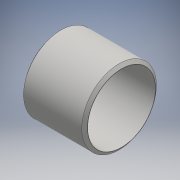
# Autodesk Inventor part: Rear Head Pipe
Saved by Autodesk Inventor 2016 (Build 200138000, 138)
## iProperties
Created: 2018-11-05
Part Number: Rear Head Pipe
Material: Steel ASTM A53 Gr.B
Document SubType Name: Modeling
Designer: asus
Density: 7.58 g/cm^3
Appearance: Plate(1)
Mass: 38975.2 g
Surface Area: 6569.07 cm^2
Volume: 5141.85 cm^3
Author: asus
Autodesk Inventor part; units mm, degrees
ref_plane "YZ Plane" through (0, 0, 0) normal (1, 0, 0) x (0, 1, 0)
ref_plane "XZ Plane" through (0, 0, 0) normal (0, 1, 0) x (-1, 0, 0)
ref_plane "XY Plane" through (0, 0, 0) normal (0, 0, 1) x (1, 0, 0)
sketch "Sketch1" plane through (0, 0, 0) normal (0, 0, 1) x (1, 0, 0)
  line L0 (-498.0346, 0) -> (498.0346, 0)
  line L1 (-138.4197, 177.8) -> (138.4197, 177.8)
  line L2 (138.4197, 177.8) -> (150, 162.7083)
  line L3 (-150, 161.1083) -> (150, 161.1083)
  line L4 (150, 161.1083) -> (150, 162.7083)
  line L5 (-150, 161.1083) -> (-150, 162.7083)
  line L6 (-150, 162.7083) -> (-138.4197, 177.8)
  point P0 (0, 0)
  point P1 (0, 0)
  point P2 (0, 177.8)
  point P3 (0, 161.1083)
  dimension "d0" = 355.6
  dimension "d1" = 322.2165
  dimension "d2" = 1.6
  dimension "d3" = 37.5
  dimension "d5" = 1.6
  dimension "d6" = 37.5
  dimension "d7" = 300
  constraints: 14 end point, 3 midpoint, 2 coincident, 2 horizontal, 2 vertical alignment, 1 perpendicular
  measures "d0" diameter of L1 L0
  measures "d1" diameter of L3 L0
  measures "d2" distance of L3.end L2.end
  measures "d3" angle of L4 L2
  measures "d5" distance of L3.start L5.end
  measures "d6" angle of L5 L6
  measures "d7" distance of L3.start L3.end
revolve "Revolution1" add sketch "Sketch1" angle 360 about axis through (-498.0346, 0, 0) along (1, 0, 0)
body "Solid1"
